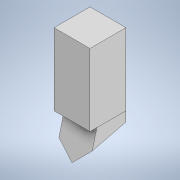
# Autodesk Inventor part: 主副偏角
Saved by Autodesk Inventor 2020 (Build 240168000, 168)
## iProperties
Created: 2020-10-11
Part Number: 主副偏角
Material: 常规
Document SubType Name: Modeling
Designer: zgz
Density: 1 g/cm^3
Appearance: 默认
Author: zgz
Autodesk Inventor part; units mm, degrees
sketch "草图1" plane through (0, 0, 0) normal (0, 0, 1) x (1, 0, 0)
  line L0 (0, 0) -> (5, 0)
  line L1 (5, 5) -> (5, 30)
  line L2 (5, 30) -> (-5, 30)
  line L3 (-5, 30) -> (-5, 2.8868)
  line L4 (-5, 0) -> (5, 0)
  line L5 (0, 0) -> (5, 5)
  line L6 (0, 0) -> (7.0711, 0) construction
  line L7 (0, 0) -> (-5, 2.8868)
  line L8 (0, 0) -> (5.7735, 0) construction
  dimension "d0" = 5
  dimension "d1" = 30
  dimension "d2" = 10
  dimension "d5" = 45
  dimension "d6" = 150
  constraints: 18 end point, 4 horizontal, 2 equal length, 2 perpendicular, 1 collinear
  measures "d0" distance of L0.start L0.end
  measures "d1" distance of L0.end L1.end
  measures "d2" distance of L1.end L2.end
  measures "d5" angle of L6 L5
  measures "d6" angle of L8 L7
extrude "拉伸1" add sketch "草图1" against normal blind 10
sketch "草图2" plane through (0, 0, 0) normal (0.7071068, -0.7071068, 0) x (-0.7071068, -0.7071068, 0)
  line L0 (0, 0) -> (-7.0711, 0) projected
  line L1 (0, 0) -> (-7.0713, 0.6187)
  line L2 (0, 0) -> (7.0983, 0) construction
  dimension "d7" = 175
  constraints: 4 end point, 1 equal length, 1 horizontal
  measures "d7" angle of L2 L1
ref_plane "工作平面4" through (-5, 10, 0) normal (0, 1, 0) x (1, 0, 0)
split body "分割1" result two bodies by plane through (-5, 10, 0) normal (0, 1, 0) first body at (1.6667, 16.6667, -0.5)
sketch3d "三维草图1"
ref_plane "副正交平面" through (0, 0, 0) normal (0.8660254, -0.5, 0) x (0.5, 0.8660254, 0)
sketch "草图4" plane through (5, 5, 0) normal (1, 0, 0) x (0, 0, -1)
  line L0 (0, 0) -> (10, 0) projected
  line L1 (0.6208, 0) -> (0.6208, 25)
  line L2 (0, 25) -> (10, 25) projected
  point P0 (0, -5)
  constraints: 2 end point, 2 point on line, 1 vertical
sketch "草图5" plane through (-5, 30, 0) normal (0, 1, 0) x (1, 0, 0)
  line L0 (5, 0) -> (10, 0.619)
  line L1 (10, 0) -> (10, 10) projected
  line L2 (10, 0) -> (0, 0) projected
  line L3 (5, 0) -> (10, 0)
  line L4 (10, 0) -> (10, 0.619)
  constraints: 6 end point, 1 collinear, 1 perpendicular, 1 point on line
extrude "拉伸2" cut sketch "草图5" against normal blind 30 bodies 3
ref_plane "正交平面2" through (0, 0, 0) normal (-0.7071068, -0.7071068, 0) x (0, 0, -1)
ref_plane "正交平面" through (5, 5, 0) normal (-0.7071068, -0.7071068, 0) x (0, 0, -1)
sketch "草图6" plane through (0, 0, 0) normal (-0.7071068, -0.7071068, 0) x (0, 0, -1)
  line L0 (0, 0) -> (0, -21.2132) projected
  line L1 (0, 0) -> (2.4419, -9.1132)
  line L2 (0, 0) -> (9.4347, 0) construction
  line L3 (0, -24.7487) -> (0, -5.5768) projected
  line L4 (0, -5.5768) -> (0, 0) projected
  line L5 (0, 0) -> (10.9149, -1.9246)
  line L6 (0, 0) -> (11.0833, 0) construction
  dimension "d11" = 75
  dimension "d18" = 10
  constraints: 9 end point, 2 equal length, 2 horizontal
  measures "d11" angle of L1 L2
  measures "d18" angle of L5 L6
sketch "草图7" plane through (-5, 2.8868, 0) normal (-1, 0, 0) x (0, 0, 1)
  point P0 (0, -2.8868)
ref_plane "工作平面3" through (0, 0, 0) normal (-0.122781, 0.2419428, 0.9624908) x (0.7044127, 0.7044127, -0.0872102)
sketch "草图8" plane through (0, 0, 0) normal (-0.122781, 0.2419428, 0.9624908) x (0.7044127, 0.7044127, -0.0872102)
  line L0 (0, 0) -> (7.0441, 6.6728) projected
  line L1 (0, 0) -> (15, 0)
  line L2 (15, 0) -> (15, 15)
  line L3 (15, 15) -> (-5, 15)
  line L4 (-5, 15) -> (-5, 0)
  line L5 (0, 0) -> (0.8721, 2.5692) projected
  line L6 (-5, 0) -> (0, 0)
  dimension "d13" = 15
  dimension "d14" = 15
  dimension "d15" = 20
  constraints: 10 end point, 3 perpendicular, 2 horizontal
  measures "d13" distance of L0.start L1.end
  measures "d14" distance of L1.end L2.end
  measures "d15" distance of L2.end L3.end
extrude "拉伸3" cut sketch "草图8" along normal blind 30 bodies 3
ref_plane "工作平面5" through (0, 0, 0) normal (-0.3968015, -0.6444766, -0.6536042) x (0.6830127, -0.6830127, 0.258819)
ref_plane "工作平面6" through (5, 5, -0.619) normal (0.6855357, -0.7070319, -0.1736281) x (-0.7044127, -0.7044127, 0.0872102)
sketch "草图9" plane through (5, 5, -0.619) normal (0.6855357, -0.7070319, -0.1736281) x (-0.7044127, -0.7044127, 0.0872102)
  line L0 (-3.1536, -1.7614) -> (-3.9393, 13.0649)
  line L1 (-3.9393, 13.0649) -> (12.5056, 12.3251)
  line L2 (12.5056, 12.3251) -> (9.2397, -2.319)
  line L3 (9.2397, -2.319) -> (-3.1536, -1.7614)
  point P0 (7.0981, 0)
  constraints: 8 end point, 1 parallel
extrude "拉伸4" cut sketch "草图9" along normal blind 10 bodies 3
sketch "草图10" plane through (0, 0, 0) normal (0.8660254, -0.5, 0) x (0.5, 0.8660254, 0)
  line L0 (0, 0) -> (1.0379, -11.8633)
  line L1 (0, 0) -> (11.9087, 0) construction
  dimension "d21" = 85
  constraints: 4 end point, 1 equal length, 1 horizontal
  measures "d21" angle of L0 L1
ref_plane "工作平面8" through (-5, 2.8868, -1.3635) normal (0.4801704, 0.8728364, 0.0871373) x (0.8428408, -0.4866144, 0.2298387)
sketch "草图11" plane through (-5, 2.8868, -1.3635) normal (0.4801704, 0.8728364, 0.0871373) x (0.8428408, -0.4866144, 0.2298387)
  line L0 (-8.1584, -1.617) -> (10.6055, -5.6683)
  line L1 (10.6055, -5.6683) -> (13.6618, 13.1312)
  line L2 (13.6618, 13.1312) -> (-7.6964, 11.7807)
  line L3 (-7.6964, 11.7807) -> (-8.1584, -1.617)
  point P0 (5.9323, 0)
  constraints: 8 end point
extrude "拉伸5" cut sketch "草图11" against normal blind 10 bodies 3
